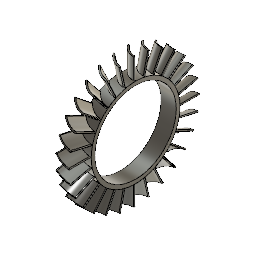
petrol_turbine_one_eng_model (Autodesk Fusion 360 design; units mm, degrees)
Autodesk Fusion 360 part; units mm, degrees
sketch "Sketch1" plane through (0, 0, 0) normal (1, 0, 0) x (0, 1, 0)
  circle A0 centre (0, 0) radius 53
  circle A1 centre (0, 0) radius 58
  dimension "d1" = 106
  dimension "d2" = 116
  constraint coincident A0.centre A1.centre
  measures "d1" diameter of A0
  measures "d2" diameter of A1
extrude "Extrude1" add sketch "Sketch1" along normal blind 20 makes body 1
sketch "Sketch2" plane through (0, 0, 0) normal (0, 0, 1) x (1, 0, 0)
  line L0 (0, 0) -> (57.1513, 0) construction
  line L1 (20, -58) -> (20, 58) construction
  line L2 (0, -58) -> (0, 58) construction
  arc A0 (0.1509, 9.4717) -> (19, -1) centre (19, 21.2) ccw
  arc A1 (1.8491, 10.5283) -> (19, 1) centre (19, 21.2) ccw
  line L3 (19, -1) -> (19, 1)
  line L4 (1.8491, 10.5283) -> (0.1509, 9.4717)
  point P0 (19, 0)
  point P1 (1, 10)
  dimension "d5" = 1
  dimension "d6" = 10
  dimension "d7" = 1
  constraint coincident L0.start origin
  constraint horizontal L0
  constraint coincident L0 P0
  constraint parallel L1 L3
  measures "d5" distance of P0 L1
  measures "d6" vertical distance of L0.start P1
  measures "d7" distance of P1 L2
extrude "Extrude2" add sketch "Sketch2" along normal blind 85 separate body makes body 2
fillet "Fillet1" radius 1 4 edges at (1.8491, 10.5283, 42.5) (19, 1, 42.5) (19, -1, 42.5) (0.1509, 9.4717, 42.5) on bodies 2
pattern_circular "C-Pattern1" count 28 over 360 about axis through (1.75, 0, 0) along (1, 0, 0) of "Extrude2", "Fillet1" makes body 3 at (14.1035, -13.0514, 55.1451) makes body 4 at (1.2946, -17.5524, 54.4425) makes body 5 at (6.1625, -32.9167, 46.2292) makes body 6 at (6.1625, -42.3783, 37.7455) makes body 7 at (3.9001, -48.9174, 29.0252) makes body 8 at (1.2946, -53.5086, 20.2213) makes body 9 at (1.2946, -56.6667, 7.8075) makes body 10 at (1.2946, -56.9833, -4.9977) makes body 11 at (3.9001, -53.1924, -20.1483) makes body 12 at (3.9001, -47.3753, -31.4795) makes body 13 at (3.9001, -39.1827, -41.2323) makes body 14 at (1.898, -30.9342, -47.9981) makes body 15 at (5.3818, -9.8805, -26.8068) makes body 16 at (6.1625, -3.0882, -56.6667) makes body 17 at (3.9001, 7.8067, -56.3421) makes body 18 at (6.1625, 21.8044, -52.3948) makes body 19 at (1.2946, 29.2269, -49.1717) makes body 20 at (6.1625, 42.3783, -37.7455) makes body 21 at (3.9001, 48.9174, -29.0252) makes body 22 at (1.2946, 53.5086, -20.2213) makes body 23 at (6.1625, 56.6667, -3.0882) makes body 24 at (6.1625, 55.9331, 9.5988) makes body 25 at (3.9001, 53.1924, 20.1483) makes body 26 at (6.1625, 46.2292, 32.9167) makes body 27 at (8.6463, 36.5525, 43.3297) makes body 28 at (1.2946, 31.6211, 47.6673) makes body 29 at (6.1625, 15.6203, 54.5587)
sketch "Sketch3" plane through (20, 0, 0) normal (1, 0, 0) x (0, 1, 0)
  circle A0 centre (0, 0) radius 53
  circle A1 centre (0, 0) radius 58
  circle A2 centre (0, 0) radius 53
  dimension "d16" = 106
  constraint coincident A0.centre A1.centre
  measures "d16" diameter of A2
extrude "Extrude3" cut sketch "Sketch3" along normal mid plane 80 contours A0 A2 bodies 2 3 4 5 6 7 8 9 10 11 12 13 14 15 16 17 18 19 20 21 22 23 24 25 26 27 28 29
combine "Combine1" operation add target body 14 tool bodies 11 10 18 9 21 8 7 22 3 15 29 2 12 17 27 6 20 16 28 13 19 24 4 26 25 23 5 1
